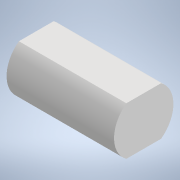
# Autodesk Inventor part: TTmotor
Saved by Autodesk Inventor 2022 (Build 260153070, 153G)
## iProperties
Created: 2021-11-29
Part Number: TTmotor
Material: Generic
Document SubType Name: Modeling
Designer: a laptop
Density: 1 g/cm^3
Appearance: Default
Author: a laptop
Autodesk Inventor part; units mm, degrees
ref_plane "YZ Plane" through (0, 0, 0) normal (1, 0, 0) x (0, 1, 0)
ref_plane "XZ Plane" through (0, 0, 0) normal (0, 1, 0) x (-1, 0, 0)
ref_plane "XY Plane" through (0, 0, 0) normal (0, 0, 1) x (1, 0, 0)
sketch "Sketch1" plane through (0, 0, 0) normal (1, 0, 0) x (0, 1, 0)
  arc A0 (7.5, 5.4141) -> (-7.5, 5.4141) centre (0, 0) ccw
  line L0 (7.5, 5.4141) -> (7.5, -5.4141)
  line L1 (-7.5, -5.4141) -> (-7.5, 5.4141)
  arc A1 (7.5, -5.4141) -> (7.5, 5.4141) centre (0, 0) ccw construction
  arc A2 (-7.5, -5.4141) -> (7.5, -5.4141) centre (0, 0) ccw
  arc A3 (-7.5, 5.4141) -> (-7.5, -5.4141) centre (0, 0) ccw construction
  line L2 (11.125, 9.25) -> (11.125, -9.25) projected
  dimension "d2" = 18.5
  dimension "d3" = 15
  constraints: 9 point on circle, 4 centre point, 4 end point, 3 parallel, 1 coincident, 1 vertical
  measures "d2" diameter of A0
  measures "d3" distance between parallel lines of L0 L1
extrude "Extrusion2" add sketch "Sketch1" along normal blind 33.5
body "Solid2"
